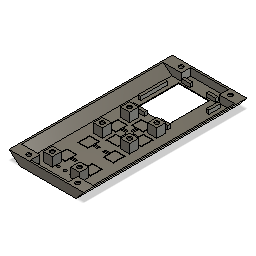
Front_Cover (Autodesk Fusion 360 design; units mm, degrees)
Autodesk Fusion 360 part; units mm, degrees
sketch "Sketch1" plane through (0, 0, 0) normal (0, 0, 1) x (1, 0, 0)
  line L0 (-6.9175, 10) -> (5, 0)
  line L1 (5, 0) -> (66.9345, 0)
  line L2 (66.9345, 0) -> (75.3255, 10)
  line L3 (75.3255, 10) -> (-6.9175, 10)
  line L4 (6.8669, 0) -> (-5.0507, 10)
  line L5 (65.368, 0) -> (73.759, 10)
  line L6 (68.6127, 2) -> (2.6165, 2)
  line L7 (15.0825, 10) -> (15.0825, 0)
  line L8 (56.8255, 10) -> (56.8255, 0)
  dimension "d1" = 140
  dimension "d2" = 130
  dimension "d4" = 82.243
  dimension "d5" = 10
  dimension "d6" = 2
  dimension "d7" = 1.2
  dimension "d8" = 1.2
  dimension "d185" = 18.5
  dimension "d186" = 22
  constraint horizontal L1
  constraint parallel L1 L3
  constraint coincident L1 L4.start
  constraint coincident L3 L4.end
  constraint parallel L0 L4
  constraint coincident L1 L5.start
  constraint coincident L3 L5.end
  constraint perpendicular L4 L5
  constraint coincident L2 L6.start
  constraint coincident L0 L6.end
  constraint parallel L1 L6
  constraint coincident L3 L7.start
  constraint coincident L1 L7.end
  constraint perpendicular L1 L7
  constraint coincident L3 L8.start
  constraint coincident L1 L8.end
  constraint perpendicular L1 L8
  measures "d1" angle of L0 L1
  measures "d2" angle of L1 L2
  measures "d4" distance of L0.start L2.end
  measures "d5" distance of L1 L3
  measures "d6" distance of L1 L6
  measures "d7" distance of L0 L4
  measures "d8" distance of L2 L5
  measures "d185" distance of L2.end L8
  measures "d186" distance of L0.start L7
extrude "Extrude1" add sketch "Sketch1" along normal blind 2
extrude "Extrude2" add sketch "Sketch1" along normal blind 176 from surface at 2 contours L0 L3 L4 L6 | L0 L1 L4 L6 | L1 L4 L6 L7 | L1 L6 L7 L8 | L1 L5 L6 L8 | L2 L3 L5 L6 | L1 L2 L5 L6
extrude "Extrude3" add sketch "Sketch1" along normal blind 2 from surface at 178
extrude "Extrude14" add sketch "Sketch1" along normal blind 12 contours L3 L4 L6 L7 | L3 L5 L6 L8
extrude "Extrude15" add sketch "Sketch1" against normal blind 12 from surface at 180 contours L3 L4 L6 L7 | L3 L5 L6 L8
sketch "Sketch2" plane through (0, 0, 0) normal (0, -1, 0) x (1, 0, 0)
  line L0 (5, 0) -> (66.9345, 0)
  line L1 (66.9345, 0) -> (66.9345, 180)
  line L2 (66.9345, 180) -> (5, 180)
  line L3 (5, 180) -> (5, 0)
  line L4 (15.0345, 15) -> (15.0345, 61.2)
  line L5 (15.0345, 61.2) -> (48.9345, 61.2)
  line L6 (48.9345, 61.2) -> (48.9345, 15)
  line L7 (48.9345, 15) -> (15.0345, 15)
  line L8 (15.9345, 70) -> (55.9345, 70)
  line L9 (55.9345, 70) -> (55.9345, 165)
  line L10 (55.9345, 165) -> (15.9345, 165)
  line L11 (15.9345, 165) -> (15.9345, 70)
  circle A0 centre (50.9345, 75) radius 1.85
  circle A1 centre (50.9345, 105) radius 1.85
  circle A2 centre (20.9345, 75) radius 1.85
  circle A3 centre (50.9345, 160) radius 1.85
  circle A4 centre (20.9345, 160) radius 1.85
  circle A5 centre (20.9345, 105) radius 1.85
  circle A6 centre (35.9345, 75) radius 1
  circle A7 centre (35.9345, 105) radius 1
  circle A8 centre (50.9345, 90) radius 1
  circle A9 centre (20.9345, 90) radius 1
  circle A10 centre (50.9345, 121) radius 1
  circle A11 centre (20.9345, 121) radius 1
  circle A12 centre (50.9345, 146) radius 1
  circle A13 centre (20.9345, 146) radius 1
  line L12 (29.9345, 71) -> (29.9345, 81)
  line L13 (29.9345, 81) -> (34.9345, 81)
  line L14 (34.9345, 81) -> (34.9345, 87)
  line L15 (29.9345, 71) -> (41.9345, 71)
  line L16 (41.9345, 71) -> (41.9345, 81)
  line L17 (41.9345, 81) -> (36.9345, 81)
  line L18 (36.9345, 81) -> (36.9345, 87)
  line L19 (34.9345, 87) -> (34.4345, 87)
  line L20 (34.4345, 87) -> (34.4345, 81.5)
  line L21 (34.4345, 81.5) -> (29.4345, 81.5)
  line L22 (29.4345, 81.5) -> (29.4345, 70.5)
  line L23 (29.4345, 70.5) -> (42.4345, 70.5)
  line L24 (42.4345, 70.5) -> (42.4345, 81.5)
  line L25 (42.4345, 81.5) -> (37.4345, 81.5)
  line L26 (37.4345, 81.5) -> (37.4345, 87)
  line L27 (37.4345, 87) -> (36.9345, 87)
  line L28 (54.9345, 84) -> (44.9345, 84)
  line L29 (44.9345, 91) -> (38.9345, 91)
  line L30 (38.9345, 91.5) -> (38.9345, 91)
  line L31 (44.4345, 83.5) -> (55.4345, 83.5)
  line L32 (38.9345, 89) -> (38.9345, 88.5)
  line L33 (44.9345, 89) -> (38.9345, 89)
  line L34 (44.4345, 88.5) -> (44.4345, 83.5)
  line L35 (44.9345, 84) -> (44.9345, 89)
  line L36 (38.9345, 88.5) -> (44.4345, 88.5)
  line L37 (44.9345, 96) -> (44.9345, 91)
  line L38 (44.4345, 96.5) -> (44.4345, 91.5)
  line L39 (54.9345, 96) -> (44.9345, 96)
  line L40 (55.4345, 96.5) -> (44.4345, 96.5)
  line L41 (55.4345, 83.5) -> (55.4345, 96.5)
  line L42 (44.4345, 91.5) -> (38.9345, 91.5)
  line L43 (54.9345, 84) -> (54.9345, 96)
  line L44 (41.9345, 109) -> (41.9345, 99)
  line L45 (34.9345, 99) -> (34.9345, 93)
  line L46 (34.4345, 93) -> (34.9345, 93)
  line L47 (42.4345, 98.5) -> (42.4345, 109.5)
  line L48 (36.9345, 93) -> (37.4345, 93)
  line L49 (36.9345, 99) -> (36.9345, 93)
  line L50 (37.4345, 98.5) -> (42.4345, 98.5)
  line L51 (41.9345, 99) -> (36.9345, 99)
  line L52 (37.4345, 93) -> (37.4345, 98.5)
  line L53 (29.9345, 99) -> (34.9345, 99)
  line L54 (29.4345, 98.5) -> (34.4345, 98.5)
  line L55 (29.9345, 109) -> (29.9345, 99)
  line L56 (29.4345, 109.5) -> (29.4345, 98.5)
  line L57 (42.4345, 109.5) -> (29.4345, 109.5)
  line L58 (34.4345, 98.5) -> (34.4345, 93)
  line L59 (41.9345, 109) -> (29.9345, 109)
  line L60 (16.9345, 96) -> (26.9345, 96)
  line L61 (26.9345, 89) -> (32.9345, 89)
  line L62 (32.9345, 88.5) -> (32.9345, 89)
  line L63 (27.4345, 96.5) -> (16.4345, 96.5)
  line L64 (32.9345, 91) -> (32.9345, 91.5)
  line L65 (26.9345, 91) -> (32.9345, 91)
  line L66 (27.4345, 91.5) -> (27.4345, 96.5)
  line L67 (26.9345, 96) -> (26.9345, 91)
  line L68 (32.9345, 91.5) -> (27.4345, 91.5)
  line L69 (26.9345, 84) -> (26.9345, 89)
  line L70 (27.4345, 83.5) -> (27.4345, 88.5)
  line L71 (16.9345, 84) -> (26.9345, 84)
  line L72 (16.4345, 83.5) -> (27.4345, 83.5)
  line L73 (16.4345, 96.5) -> (16.4345, 83.5)
  line L74 (27.4345, 88.5) -> (32.9345, 88.5)
  line L75 (16.9345, 96) -> (16.9345, 84)
  line L76 (16.9345, 127) -> (26.9345, 127)
  line L77 (27.4345, 127.5) -> (16.4345, 127.5)
  line L78 (32.9345, 122.5) -> (27.4345, 122.5)
  line L79 (26.9345, 115) -> (26.9345, 120)
  line L80 (26.9345, 127) -> (26.9345, 122)
  line L81 (32.9345, 119.5) -> (32.9345, 120)
  line L82 (26.9345, 122) -> (32.9345, 122)
  line L83 (16.4345, 114.5) -> (27.4345, 114.5)
  line L84 (27.4345, 114.5) -> (27.4345, 119.5)
  line L85 (16.4345, 127.5) -> (16.4345, 114.5)
  circle A14 centre (20.9345, 121) radius 1
  line L86 (16.9345, 127) -> (16.9345, 115)
  line L87 (27.4345, 119.5) -> (32.9345, 119.5)
  line L88 (27.4345, 122.5) -> (27.4345, 127.5)
  line L89 (16.9345, 115) -> (26.9345, 115)
  line L90 (32.9345, 122) -> (32.9345, 122.5)
  line L91 (26.9345, 120) -> (32.9345, 120)
  circle A15 centre (50.9345, 121) radius 1
  line L92 (55.4345, 114.5) -> (55.4345, 127.5)
  line L93 (44.9345, 122) -> (38.9345, 122)
  line L94 (38.9345, 122.5) -> (38.9345, 122)
  line L95 (38.9345, 120) -> (38.9345, 119.5)
  line L96 (44.9345, 115) -> (44.9345, 120)
  line L97 (54.9345, 127) -> (44.9345, 127)
  line L98 (44.4345, 114.5) -> (55.4345, 114.5)
  line L99 (54.9345, 115) -> (54.9345, 127)
  line L100 (38.9345, 119.5) -> (44.4345, 119.5)
  line L101 (55.4345, 127.5) -> (44.4345, 127.5)
  line L102 (54.9345, 115) -> (44.9345, 115)
  line L103 (44.9345, 127) -> (44.9345, 122)
  line L104 (44.4345, 122.5) -> (38.9345, 122.5)
  line L105 (44.4345, 119.5) -> (44.4345, 114.5)
  line L106 (44.4345, 127.5) -> (44.4345, 122.5)
  circle A16 centre (50.9345, 121) radius 1
  circle A17 centre (50.9345, 121) radius 1
  line L107 (44.9345, 120) -> (38.9345, 120)
  line L108 (44.4345, 147.5) -> (38.9345, 147.5)
  line L109 (44.9345, 152) -> (44.9345, 147)
  line L110 (44.9345, 145) -> (38.9345, 145)
  line L111 (32.9345, 147.5) -> (27.4345, 147.5)
  line L112 (16.4345, 152.5) -> (16.4345, 139.5)
  line L113 (44.9345, 140) -> (44.9345, 145)
  circle A18 centre (20.9345, 146) radius 1
  line L114 (54.9345, 140) -> (44.9345, 140)
  line L115 (16.9345, 140) -> (26.9345, 140)
  circle A19 centre (50.9345, 146) radius 1
  line L116 (16.9345, 152) -> (16.9345, 140)
  line L117 (27.4345, 139.5) -> (27.4345, 144.5)
  line L118 (38.9345, 144.5) -> (44.4345, 144.5)
  line L119 (16.4345, 139.5) -> (27.4345, 139.5)
  line L120 (32.9345, 144.5) -> (32.9345, 145)
  line L121 (44.9345, 147) -> (38.9345, 147)
  circle A20 centre (20.9345, 146) radius 1
  line L122 (54.9345, 140) -> (54.9345, 152)
  line L123 (26.9345, 152) -> (26.9345, 147)
  line L124 (55.4345, 152.5) -> (44.4345, 152.5)
  line L125 (27.4345, 147.5) -> (27.4345, 152.5)
  line L126 (38.9345, 147.5) -> (38.9345, 147)
  circle A21 centre (50.9345, 146) radius 1
  line L127 (38.9345, 145) -> (38.9345, 144.5)
  line L128 (32.9345, 147) -> (32.9345, 147.5)
  line L129 (27.4345, 152.5) -> (16.4345, 152.5)
  circle A22 centre (20.9345, 146) radius 1
  circle A23 centre (50.9345, 146) radius 1
  line L130 (26.9345, 147) -> (32.9345, 147)
  line L131 (26.9345, 145) -> (32.9345, 145)
  line L132 (27.4345, 144.5) -> (32.9345, 144.5)
  circle A24 centre (53.6081, 143.5467) radius 1
  line L133 (16.9345, 152) -> (26.9345, 152)
  line L134 (26.9345, 140) -> (26.9345, 145)
  line L135 (44.4345, 139.5) -> (55.4345, 139.5)
  line L136 (44.4345, 152.5) -> (44.4345, 147.5)
  line L137 (44.4345, 144.5) -> (44.4345, 139.5)
  line L138 (55.4345, 139.5) -> (55.4345, 152.5)
  line L139 (54.9345, 152) -> (44.9345, 152)
  line L140 (34.9345, 87) -> (36.9345, 87)
  line L141 (34.9345, 81) -> (36.9345, 81)
  line L142 (44.9345, 89) -> (44.9345, 91)
  line L143 (38.9345, 89) -> (38.9345, 91)
  line L144 (36.9345, 99) -> (34.9345, 99)
  line L145 (36.9345, 93) -> (34.9345, 93)
  line L146 (26.9345, 91) -> (26.9345, 89)
  line L147 (32.9345, 91) -> (32.9345, 89)
  line L148 (26.9345, 122) -> (26.9345, 120)
  line L149 (32.9345, 122) -> (32.9345, 120)
  line L150 (44.9345, 122) -> (44.9345, 120)
  line L151 (38.9345, 120) -> (38.9345, 122)
  line L152 (26.9345, 145) -> (26.9345, 147)
  line L153 (32.9345, 147) -> (32.9345, 145)
  line L154 (38.9345, 147) -> (38.9345, 145)
  line L155 (44.9345, 145) -> (44.9345, 147)
  line L156 (25.9345, 70) -> (25.9345, 80)
  line L157 (25.9345, 80) -> (15.9345, 80)
  line L158 (15.9345, 110) -> (25.9345, 110)
  line L159 (25.9345, 110) -> (25.9345, 100)
  line L160 (25.9345, 100) -> (15.9345, 100)
  line L161 (55.9345, 110) -> (45.9345, 110)
  line L162 (45.9345, 110) -> (45.9345, 100)
  line L163 (45.9345, 100) -> (55.9345, 100)
  line L164 (45.9345, 70) -> (45.9345, 80)
  line L165 (45.9345, 80) -> (55.9345, 80)
  line L166 (45.9345, 165) -> (45.9345, 155)
  line L167 (45.9345, 155) -> (55.9345, 155)
  line L168 (15.9345, 155) -> (25.9345, 155)
  line L169 (25.9345, 155) -> (25.9345, 165)
  circle A25 centre (62.9345, 6) radius 3
  circle A26 centre (62.9345, 6) radius 1.85
  line L170 (5, 0) -> (66.9345, 0)
  circle A27 centre (8.9345, 6) radius 3
  circle A28 centre (8.9345, 6) radius 1.85
  circle A29 centre (62.9345, 174) radius 3
  circle A30 centre (62.9345, 174) radius 1.85
  circle A31 centre (8.9345, 174) radius 3
  circle A32 centre (8.9345, 174) radius 1.85
  line L171 (15, 0) -> (15, 12)
  line L172 (15, 12) -> (5, 12)
  line L173 (66.9345, 12) -> (56.9345, 12)
  line L174 (56.9345, 12) -> (56.9345, 0)
  line L175 (56.9345, 180) -> (56.9345, 168)
  line L176 (56.9345, 168) -> (66.9345, 168)
  line L177 (15, 180) -> (15, 168)
  line L178 (15, 168) -> (5, 168)
  line L179 (75.3255, 0) -> (75.3255, 180)
  circle A33 centre (43.4345, 161) radius 1.65
  circle A34 centre (35.9345, 161) radius 1.65
  circle A35 centre (28.4345, 161) radius 1.65
  line L180 (11.0345, 13.4) -> (11.0345, 62.8)
  line L181 (11.0345, 62.8) -> (58.8345, 62.8)
  line L182 (58.8345, 62.8) -> (58.8345, 13.4)
  line L183 (58.8345, 13.4) -> (11.0345, 13.4)
  line L184 (8.0345, 23.4) -> (11.0345, 23.4)
  line L185 (8.0345, 52.8) -> (11.0345, 52.8)
  line L186 (8.0345, 52.8) -> (8.0345, 23.4)
  line L187 (43.8345, 62.8) -> (43.8345, 65.8)
  line L188 (43.8345, 65.8) -> (53.8345, 65.8)
  line L189 (53.8345, 65.8) -> (53.8345, 62.8)
  line L190 (43.8345, 13.4) -> (43.8345, 10.4)
  line L191 (43.8345, 10.4) -> (53.8345, 10.4)
  line L192 (53.8345, 10.4) -> (53.8345, 13.4)
  line L193 (58.8345, 28.4) -> (61.8345, 28.4)
  line L194 (61.8345, 28.4) -> (61.8345, 15.4)
  line L195 (61.8345, 15.4) -> (58.8345, 15.4)
  line L196 (25.4417, 142.5872) -> (25.4417, 149.4182) construction
  line L197 (25.4417, 149.4182) -> (15.4417, 149.4182) construction
  line L198 (15.4417, 149.4182) -> (15.4417, 142.5872) construction
  line L199 (15.4417, 142.5872) -> (25.4417, 142.5872) construction
  line L200 (53.6081, 143.5467) -> (53.6081, 149.8553) construction
  line L201 (53.6081, 149.8553) -> (43.6081, 149.8553) construction
  line L202 (43.6081, 149.8553) -> (43.6081, 143.5467) construction
  line L203 (43.6081, 143.5467) -> (53.6081, 143.5467) construction
  line L204 (23.9421, 92.4236) -> (19.2009, 92.4236) construction
  line L205 (19.2009, 92.4236) -> (19.2009, 82.4236) construction
  line L206 (19.2009, 82.4236) -> (23.9421, 82.4236) construction
  line L207 (23.9421, 82.4236) -> (23.9421, 92.4236) construction
  line L208 (47.7311, 87.5657) -> (52.4724, 87.5657) construction
  line L209 (52.4724, 87.5657) -> (52.4724, 97.5657) construction
  line L210 (52.4724, 97.5657) -> (47.7311, 97.5657) construction
  line L211 (47.7311, 97.5657) -> (47.7311, 87.5657) construction
  line L212 (33.4966, 78.2323) -> (33.4966, 73.4911) construction
  line L213 (33.4966, 73.4911) -> (43.4966, 73.4911) construction
  line L214 (43.4966, 73.4911) -> (43.4966, 78.2323) construction
  line L215 (43.4966, 78.2323) -> (33.4966, 78.2323) construction
  line L216 (38.3759, 101.7527) -> (38.3759, 106.4939) construction
  line L217 (38.3759, 106.4939) -> (28.3759, 106.4939) construction
  line L218 (28.3759, 106.4939) -> (28.3759, 101.7527) construction
  line L219 (28.3759, 101.7527) -> (38.3759, 101.7527) construction
  line L220 (25.4927, 118.5136) -> (25.4927, 123.8554) construction
  line L221 (25.4927, 123.8554) -> (15.4927, 123.8554) construction
  line L222 (15.4927, 123.8554) -> (15.4927, 118.5136) construction
  line L223 (15.4927, 118.5136) -> (25.4927, 118.5136) construction
  line L224 (53.5329, 117.9984) -> (53.5329, 124.5609) construction
  line L225 (53.5329, 124.5609) -> (43.5329, 124.5609) construction
  line L226 (43.5329, 124.5609) -> (43.5329, 117.9984) construction
  line L227 (43.5329, 117.9984) -> (53.5329, 117.9984) construction
  line L228 (30.7602, 165.0681) -> (30.7602, 169.8498) construction
  line L229 (30.7602, 169.8498) -> (23.7602, 169.8498) construction
  line L230 (23.7602, 169.8498) -> (23.7602, 165.0681) construction
  line L231 (23.7602, 165.0681) -> (30.7602, 165.0681) construction
  line L232 (38.889, 165.4328) -> (38.889, 169.4215) construction
  line L233 (38.889, 169.4215) -> (31.889, 169.4215) construction
  line L234 (31.889, 169.4215) -> (31.889, 165.4328) construction
  line L235 (31.889, 165.4328) -> (38.889, 165.4328) construction
  line L236 (46.0968, 167.2408) -> (46.0968, 167.9039) construction
  line L237 (46.0968, 167.9039) -> (39.0968, 167.9039) construction
  line L238 (39.0968, 167.9039) -> (39.0968, 167.2408) construction
  line L239 (39.0968, 167.2408) -> (46.0968, 167.2408) construction
  line L240 (43.8345, 65.8) -> (43.8345, 62.8)
  line L241 (28.0345, 62.8) -> (28.0345, 65.8)
  line L242 (28.0345, 65.8) -> (13.0345, 65.8)
  line L243 (13.0345, 65.8) -> (13.0345, 62.8)
  line L244 (26.0345, 13.4) -> (26.0345, 10.4)
  line L245 (26.0345, 10.4) -> (17.0345, 10.4)
  line L246 (17.0345, 10.4) -> (17.0345, 13.4)
  point P0 (35.9345, 90)
  point P1 (35.9345, 121)
  point P2 (35.9345, 146)
  point P3 (35.9345, 146)
  point P4 (20.9345, 121)
  dimension "d17" = 46.2
  dimension "d18" = 33.9
  dimension "d19" = 18
  dimension "d20" = 95
  dimension "d21" = 165
  dimension "d22" = 15
  dimension "d23" = 40
  dimension "d24" = 11
  dimension "d25" = 3.7
  dimension "d26" = 3.7
  dimension "d29" = -30
  dimension "d30" = 85
  dimension "d31" = 5
  dimension "d32" = 5
  dimension "d33" = 5
  dimension "d34" = 30
  dimension "d37" = -30
  dimension "d38" = 0
  dimension "d41" = 2
  dimension "d42" = 20
  dimension "d43" = 5
  dimension "d46" = 0
  dimension "d47" = 30
  dimension "d48" = 5
  dimension "d49" = 20
  dimension "d50" = 2
  dimension "d53" = -30
  dimension "d54" = 0
  dimension "d55" = 2
  dimension "d56" = 5
  dimension "d57" = 51
  dimension "d60" = -30
  dimension "d61" = 25
  dimension "d62" = 12
  dimension "d63" = 6
  dimension "d64" = 10
  dimension "d65" = 10
  dimension "d66" = 4
  dimension "d67" = 1
  dimension "d68" = 1
  dimension "d70" = 6
  dimension "d71" = 0.5
  dimension "d72" = 0.5
  dimension "d73" = 0.5
  dimension "d74" = 0.5
  dimension "d75" = 0.5
  dimension "d76" = 0.5
  dimension "d77" = 0.5
  dimension "d79" = 360
  dimension "d92" = 20
  dimension "d93" = 20
  dimension "d94" = 20
  dimension "d95" = 20
  dimension "d96" = 25
  dimension "d97" = 31
  dimension "d101" = 10
  dimension "d102" = 10
  dimension "d103" = 10
  dimension "d104" = 10
  dimension "d105" = 10
  dimension "d106" = 10
  dimension "d107" = 5
  dimension "d108" = 10
  dimension "d109" = 10
  dimension "d110" = 5
  dimension "d111" = 10
  dimension "d112" = 10
  dimension "d113" = 10
  dimension "d114" = 10
  dimension "d118" = 6
  dimension "d119" = 3.7
  dimension "d120" = 6
  dimension "d121" = 4
  dimension "d125" = -54
  dimension "d126" = 168
  dimension "d127" = 12
  dimension "d128" = 10
  dimension "d129" = 12
  dimension "d130" = 10
  dimension "d131" = 12
  dimension "d132" = 10
  dimension "d133" = 10
  dimension "d134" = 12
  dimension "d139" = 12.391
  dimension "d140" = 3.3
  dimension "d141" = 12.5
  dimension "d142" = 91
  dimension "d145" = -7.5
  dimension "d146" = 0
  dimension "d150" = 49.4
  dimension "d151" = 47.8
  dimension "d152" = 1.6
  dimension "d153" = 4
  dimension "d154" = 10
  dimension "d155" = 10
  dimension "d156" = 3
  dimension "d157" = 3
  dimension "d159" = 5
  dimension "d160" = 3
  dimension "d162" = 5
  dimension "d166" = 3
  dimension "d167" = 2
  dimension "d172" = 3
  dimension "d173" = 2
  dimension "d174" = 15
  dimension "d176" = 10
  dimension "d177" = 10
  dimension "d178" = 3
  dimension "d179" = 15
  dimension "d180" = 6
  dimension "d181" = 15
  text T0 "M" font "Arial" height 10 align ink ink in box 0 x 0 at (25.4417, 142.5872) x (0, 1) y (-1, 0) spacing 1 height is em
  text T1 "R" font "Arial" height 10 align ink ink in box 0 x 0 at (53.6081, 143.5467) x (0, 1) y (-1, 0) spacing 1 height is em
  text T2 ">" font "Arial" height 10 align ink ink in box 0 x 0 at (23.9421, 92.4236) x (-1, 0) y (0, -1) spacing 1 height is em
  text T3 ">" font "Arial" height 10 align ink ink in box 0 x 0 at (47.7311, 87.5657) x (1, 0) y (0, 1) spacing 1 height is em
  text T4 ">" font "Arial" height 10 align ink ink in box 0 x 0 at (33.4966, 78.2323) x (0, -1) y (1, 0) spacing 1 height is em
  text T5 ">" font "Arial" height 10 align ink ink in box 0 x 0 at (38.3759, 101.7527) x (0, 1) y (-1, 0) spacing 1 height is em
  text T6 "E" font "Arial" height 10 align ink ink in box 0 x 0 at (25.4927, 118.5136) x (0, 1) y (-1, 0) spacing 1 height is em
  text T7 "X" font "Arial" height 10 align ink ink in box 0 x 0 at (53.5329, 117.9984) x (0, 1) y (-1, 0) spacing 1 height is em
  text T8 "M" font "Arial" height 7 align ink ink in box 0 x 0 at (30.7602, 165.0681) x (0, 1) y (-1, 0) spacing 1 height is em
  text T9 "S" font "Arial" height 7 align ink ink in box 0 x 0 at (38.889, 165.4328) x (0, 1) y (-1, 0) spacing 1 height is em
  text T10 "I" font "Arial" height 7 align ink ink in box 0 x 0 at (46.0968, 167.2408) x (0, 1) y (-1, 0) spacing 1 height is em
  constraint vertical L4
  constraint perpendicular L4 L5
  constraint perpendicular L5 L6
  constraint perpendicular L6 L7
  constraint horizontal L8
  constraint perpendicular L8 L9
  constraint perpendicular L9 L10
  constraint perpendicular L8 L11
  constraint vertical L12
  constraint perpendicular L12 L13
  constraint perpendicular L13 L14
  constraint perpendicular L12 L15
  constraint perpendicular L15 L16
  constraint perpendicular L12 L17
  constraint perpendicular L17 L18
  constraint perpendicular L14 L19
  constraint perpendicular L19 L20
  constraint perpendicular L14 L21
  constraint perpendicular L19 L22
  constraint perpendicular L14 L23
  constraint perpendicular L23 L24
  constraint perpendicular L24 L25
  constraint perpendicular L25 L26
  constraint parallel L19 L27
  constraint equal L14 L18
  constraint perpendicular L107 L150
  constraint perpendicular L93 L151
  constraint perpendicular L130 L152
  constraint perpendicular L131 L153
  constraint perpendicular L110 L154
  constraint perpendicular L121 L155
  constraint coincident L8 L156.start
  constraint perpendicular L8 L156
  constraint perpendicular L156 L157
  constraint coincident L11 L157.end
  constraint coincident L11 L158.start
  constraint perpendicular L11 L158
  constraint perpendicular L158 L159
  constraint coincident L11 L160.end
  constraint perpendicular L11 L160
  constraint coincident L9 L161.start
  constraint perpendicular L9 L161
  constraint perpendicular L161 L162
  constraint coincident L9 L163.end
  constraint perpendicular L9 L163
  constraint coincident L8 L164.start
  constraint perpendicular L8 L164
  constraint coincident L9 L165.end
  constraint perpendicular L9 L165
  constraint coincident L10 L166.start
  constraint perpendicular L10 L166
  constraint coincident L9 L167.end
  constraint perpendicular L9 L167
  constraint perpendicular L9 L168
  constraint coincident L10 L169.end
  constraint perpendicular L10 L169
  constraint coincident L11 L168.start
  constraint concentric A25 A26
  constraint coincident L170 L171.start
  constraint perpendicular L170 L171
  constraint coincident L3 L172.end
  constraint perpendicular L3 L172
  constraint coincident L1 L173.start
  constraint perpendicular L1 L173
  constraint coincident L0 L174.end
  constraint perpendicular L0 L174
  constraint coincident L2 L175.start
  constraint perpendicular L2 L175
  constraint coincident L1 L176.end
  constraint perpendicular L1 L176
  constraint coincident L2 L177.start
  constraint perpendicular L2 L177
  constraint coincident L3 L178.end
  constraint perpendicular L3 L178
  constraint perpendicular L7 L180
  constraint perpendicular L180 L181
  constraint perpendicular L181 L182
  constraint perpendicular L180 L183
  constraint coincident L180 L184.end
  constraint perpendicular L180 L184
  constraint coincident L180 L185.end
  constraint perpendicular L180 L185
  constraint perpendicular L184 L186
  constraint coincident L181 L187.start
  constraint perpendicular L181 L187
  constraint perpendicular L187 L188
  constraint coincident L181 L189.end
  constraint perpendicular L181 L189
  constraint coincident L183 L190.start
  constraint perpendicular L183 L190
  constraint perpendicular L190 L191
  constraint coincident L183 L192.end
  constraint perpendicular L183 L192
  constraint coincident L182 L193.start
  constraint perpendicular L182 L193
  constraint perpendicular L193 L194
  constraint coincident L182 L195.end
  constraint perpendicular L182 L195
  constraint perpendicular L196 L197
  constraint parallel L196 L198
  constraint parallel L197 L199
  constraint perpendicular L200 L201
  constraint parallel L200 L202
  constraint parallel L201 L203
  constraint coincident A24.centre L200.start
  constraint perpendicular L204 L205
  constraint parallel L204 L206
  constraint parallel L205 L207
  constraint perpendicular L208 L209
  constraint parallel L208 L210
  constraint parallel L209 L211
  constraint perpendicular L212 L213
  constraint parallel L212 L214
  constraint parallel L213 L215
  constraint perpendicular L216 L217
  constraint parallel L216 L218
  constraint parallel L217 L219
  constraint perpendicular L220 L221
  constraint parallel L220 L222
  constraint parallel L221 L223
  constraint perpendicular L224 L225
  constraint parallel L224 L226
  constraint parallel L225 L227
  constraint perpendicular L228 L229
  constraint parallel L228 L230
  constraint parallel L229 L231
  constraint perpendicular L232 L233
  constraint parallel L232 L234
  constraint parallel L233 L235
  constraint perpendicular L236 L237
  constraint parallel L236 L238
  constraint parallel L237 L239
  constraint coincident L181 L241.start
  constraint perpendicular L181 L241
  constraint perpendicular L4 L242
  constraint coincident L181 L243.end
  constraint perpendicular L181 L243
  constraint coincident L183 L244.start
  constraint perpendicular L183 L244
  constraint perpendicular L244 L245
  constraint coincident L183 L246.end
  constraint perpendicular L183 L246
  measures "d17" distance of L5 L7
  measures "d18" distance of L4 L6
  measures "d19" distance of L1 L6
  measures "d20" distance of L8 L10
  measures "d21" distance of L2 L7
  measures "d22" distance of L2 L10
  measures "d23" distance of L9 L11
  measures "d24" distance of L1 L9
  measures "d25" diameter of A1
  measures "d26" diameter of A0
  measures "d31" distance of L9 A0.centre
  measures "d32" distance of L8 A0.centre
  measures "d33" distance of L9 A1.centre
  measures "d34" distance of A0.centre A1.centre
  measures "d41" diameter of A6
  measures "d42" distance of L9 A6.centre
  measures "d43" distance of L8 A6.centre
  measures "d48" distance of L9 A8.centre
  measures "d49" distance of L8 A8.centre
  measures "d50" diameter of A8
  measures "d55" diameter of A10
  measures "d56" distance of L9 A10.centre
  measures "d57" distance of L8 A10.centre
  measures "d62" distance of L12 L16
  measures "d63" distance of A6.centre L16
  measures "d64" distance of L15 L17
  measures "d65" distance of L13 L15
  measures "d66" distance of A6.centre L15
  measures "d67" distance of A6.centre L18
  measures "d68" distance of A6.centre L14
  measures "d70" distance of L13 L14.end
  measures "d71" distance of L18 L26
  measures "d72" distance of L17 L25
  measures "d73" distance of L14 L20
  measures "d74" distance of L13 L21
  measures "d75" distance of L12 L22
  measures "d76" distance of L15 L23
  measures "d77" distance of L16 L24
  measures "d92" distance of L8 P0
  measures "d93" distance of L9 P0
  measures "d94" distance of L9 P1
  measures "d95" distance of L9 P3
  measures "d96" distance of P1 P3
  measures "d97" distance of P0 P1
  measures "d101" distance of L8 L157
  measures "d102" distance of L11 L156
  measures "d103" distance of L10 L168
  measures "d104" distance of L11 L169
  measures "d105" distance of L9 L166
  measures "d106" distance of L10 L167
  measures "d107" distance of A1.centre L161
  measures "d108" distance of L161 L163
  measures "d109" distance of L9 L162
  measures "d110" distance of A5.centre L158
  measures "d111" distance of L158 L160
  measures "d112" distance of L11 L159
  measures "d113" distance of L8 L165
  measures "d114" distance of L9 L164
  measures "d118" diameter of A25
  measures "d119" diameter of A26
  measures "d120" distance of A25.centre L170
  measures "d121" distance of L1 A25.centre
  measures "d127" distance of L2 L178
  measures "d128" distance of L3 L177
  measures "d129" distance of L170 L172
  measures "d130" distance of L3 L171
  measures "d131" distance of L170 L173
  measures "d132" distance of L1 L174
  measures "d133" distance of L1 L175
  measures "d134" distance of L2 L176
  measures "d139" distance of A29.centre L179
  measures "d140" diameter of A33
  measures "d141" distance of L9 A33.centre
  measures "d142" distance of L8 A33.centre
  measures "d150" distance of L181 L183
  measures "d151" distance of L180 L182
  measures "d152" distance of L7 L183
  measures "d153" distance of L4 L180
  measures "d154" distance of L183 L184
  measures "d155" distance of L181 L185
  measures "d156" distance of L180 L186
  measures "d157" distance of L181 L188
  measures "d159" distance of L182 L189
  measures "d160" distance of L183 L191
  measures "d162" distance of L182 L192
  measures "d166" distance of L182 L194
  measures "d167" distance of L183 L195
  measures "d172" distance of L181 L242
  measures "d173" distance of L180 L243
  measures "d174" distance of L241 L243
  measures "d176" distance of L190 L192
  measures "d177" distance of L187 L189
  measures "d178" distance of L183 L245
  measures "d179" distance of L183 L193
  measures "d180" distance of L180 L246
  measures "d181" distance of L180 L244
extrude "Extrude4" cut sketch "Sketch2" against normal blind 15 contours L4 L5 L6 L7
extrude "Extrude5" cut sketch "Sketch2" against normal blind 5 contours L12 L13 L14 L15 L16 L17 L18 L19 L20 L21 L22 L23 L24 L25 L26 L27 | L28 L29 L30 L31 L32 L33 L34 L35 L36 L37 L38 L39 L40 L41 L42 L43 | L44 L45 L46 L47 L48 L49 L50 L51 L52 L53 L54 L55 L56 L57 L58 L59 | L60 L61 L62 L63 L64 L65 L66 L67 L68 L69 L70 L71 L72 L73 L74 L75 | L76 L77 L78 L79 L80 L81 L82 L83 L84 L85 L86 L87 L88 L89 L90 L91 | L92 L93 L94 L95 L96 L97 L98 L99 L100 L101 L102 L103 L104 L105 L106 L107 | L108 L109 L110 L113 L114 L118 L121 L122 L124 L126 L127 L135 L136 L137 L138 L139 | L111 L112 L115 L116 L117 L119 L120 L123 L125 L128 L129 L130 L131 L132 L133 L134
extrude "Extrude6" cut sketch "Sketch2" along normal blind 1 from surface at -2 contours L14 L18 L140 L141 | L29 L33 L142 L143 | L45 L49 L144 L145 | L61 L65 L146 L147 | L82 L91 L148 L149 | L93 L107 L150 L151 | L110 L121 L154 L155 | L130 L131 L152 L153
extrude "Extrude7" add sketch "Sketch2" against normal blind 10 from surface at -2 contours L8 L11 L156 L157 | L8 L9 L164 L165 | L11 L158 L159 L160 | L10 L11 L168 L169 | L9 L161 L162 L163 | L9 L10 L166 L167
extrude "Extrude8" cut sketch "Sketch2" against normal blind 15 contours A26 | A28 | A30 | A32
extrude "Extrude9" cut sketch "Sketch2" against normal blind 3.5 contours A25 | A26 | A27 | A28 | A29 | A30 | A31 | A32
extrude "Extrude10" cut sketch "Sketch2" against normal blind 5 contours A33 | A34 | A35
chamfer "Chamfer1" distance 1.2 angle 45 4 edges at (31.9845, 0, 15) (15.0345, 0, 38.1) (31.9845, 0, 61.2) (48.9345, 0, 38.1)
extrude "Extrude11" add sketch "Sketch2" against normal blind 4 from surface at -2 contours L180 L184 L185 L186 | L183 L244 L245 L246 | L183 L190 L191 L192 | L181 L241 L242 L243 | L181 L187 L188 L189 L240 | L182 L193 L194 L195
extrude "Extrude12" cut sketch "Sketch2" against normal blind 0.5 text T6 T0 T1 T7 T3 T5 T2 T4 T8 T9 T10
extrude "Extrude13" add sketch "Sketch2" against normal blind 0.2 from surface at -3.5 contours A25 | A26 | A27 | A28 | A29 | A30 | A31 | A32
chamfer "Chamfer2" distance 0.6 angle 45 10 edges at (61.2097, 10, 173.331) (49.2097, 12, 159.331) (49.2097, 12, 104.331) (49.2097, 12, 74.331) (61.2097, 10, 5.331) (7.2097, 10, 5.331) (19.2097, 12, 74.331) (19.2097, 12, 104.331) (19.2097, 12, 159.331) (7.2097, 10, 173.331)
